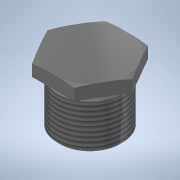
# Autodesk Inventor part: Korek sześciokątny BSP 3/4'' L=26
Saved by Autodesk Inventor 2020 (Build 240168000, 168)
## iProperties
RuleStatus: InUse
Created: 2022-03-21
Part Number: Korek sześciokątny BSP 3/4'' L=26
Material: 304
Description: Korek sześciokątny BSP 3/4'' L=26
Document SubType Name: Modelowanie
Designer: Radosław
Density: 8 g/cm^3
Sheet Metal Rule: 1,5
Sheet Metal Width: 0,000 mm
Sheet Metal Length: 0,000 mm
Sheet Metal Area: 0,000 mm^2
Appearance: Częściowo polerowany(1)
Author: Radosław
Autodesk Inventor part; units mm, degrees
ref_plane "YZ Plane" through (0, 0, 0) normal (1, 0, 0) x (0, 1, 0)
ref_plane "XZ Plane" through (0, 0, 0) normal (0, 1, 0) x (-1, 0, 0)
ref_plane "XY Plane" through (0, 0, 0) normal (0, 0, 1) x (1, 0, 0)
sketch "Szkic7" plane through (0, 0, 0) normal (0, 0, 1) x (1, 0, 0)
  circle A0 centre (0, 0) radius 13.2205
  dimension "d35" = 26.441
  constraints: 1 centre point, 1 coincident
  measures "d35" diameter of A0
extrude "Wyciągnięcie proste2" add sketch "Szkic7" along normal mid plane 19.175
chamfer "Faza2" distance 1 angle 45 1 edges at (-13.2205, 0, 9.5875)
sketch "Szkic9" plane through (0, 0, 9.5875) normal (0, 0, 1) x (1, 0, 0)
  circle A0 centre (0, 0) radius 12.2205 projected
extrude "Wyciągnięcie proste3" add sketch "Szkic9" along normal blind 1.625
sketch "Szkic10" plane through (0, 0, 11.2125) normal (0, 0, 1) x (1, 0, 0)
  line L0 (-8.6603, 15) -> (8.6603, 15)
  line L1 (8.6603, 15) -> (17.3205, 0)
  line L2 (17.3205, 0) -> (8.6603, -15)
  line L3 (8.6603, -15) -> (-8.6603, -15)
  line L4 (-8.6603, -15) -> (-17.3205, 0)
  line L5 (-17.3205, 0) -> (-8.6603, 15)
  line L6 (0, 18.5087) -> (0, -18.5087) construction
  line L7 (-18.5087, 0) -> (18.5087, 0) construction
  point P0 (0, 0)
  point P1 (0, 0)
  point P2 (0, 15)
  dimension "d44" = 30
  constraints: 12 end point, 2 point on line, 1 coincident, 1 midpoint, 13 other
  measures "d44" distance between parallel lines of L4 L1
extrude "Wyciągnięcie proste4" add sketch "Szkic10" along normal blind 5.2
sketch "Szkic12" plane through (0, 0, 0) normal (0, 1, 0) x (-1, 0, 0)
  line L0 (0, -2.1463) -> (0, 12.8775) construction
  line L1 (-8.6603, 11.2125) -> (-8.6603, 16.4125) construction
  line L2 (-17.3205, 16.4125) -> (-8.6603, 16.4125) construction
  line L3 (-17.3205, 11.2125) -> (-17.3205, 16.4125) projected
  line L4 (-17.3205, 15.8766) -> (-15.3205, 16.4125)
  line L5 (-17.3205, 16.4125) -> (-8.6603, 16.4125) projected
  line L6 (-17.3205, 11.2125) -> (-8.6603, 11.2125) projected
  point P0 (0, 0)
  dimension "d50" = 15
  dimension "d51" = 2
  constraints: 2 end point, 2 point on line
  measures "d50" angle of L2 L4
  measures "d51" distance from line of L3 L4.end
revolve "Obrót2" cut sketch "Szkic12" angle 360 about axis through (0, 0, -10) along (0, 0, 1)
thread "Gwint3" size "G26.441x1.814" designation "G 3/4" class "A" standard "ISO Pipe Threads" full length
chamfer "Faza3" distance 1 angle 45 1 edges at (-13.2205, 0, -9.5875)
equation "\"d35\" = OD"
equation "\"d36\" = 0.7375 * L"
equation "\"d42\" = 0.0625 * L"
equation "\"d44\" = SW"
equation "\"d45\" = 0.2 * L"
equation "\"d51\" = 0.0666667 * SW"
equation "\"SzerokośćGięciaPodcięcia\" = Grubość"
equation "\"RozmiarPodcięciaNarożnika\" = 4 * Grubość"
equation "\"PromieńPrzejścia\" = PromieńGięcia"
equation "\"Rozmiar_promienia_Jacobiego\" = PromieńGięcia"
equation "\"Wielk_odstępu\" = Grubość"
equation "\"d2\" = PromieńGięcia"
equation "\"d23\" = PromieńGięcia"
equation "\"OD\" = 26.441"
equation "\"SW\" = 30"
equation "\"L\" = 26"
equation "\"Grubość\" = 1.5"
equation "\"PromieńGięcia\" = 3"
